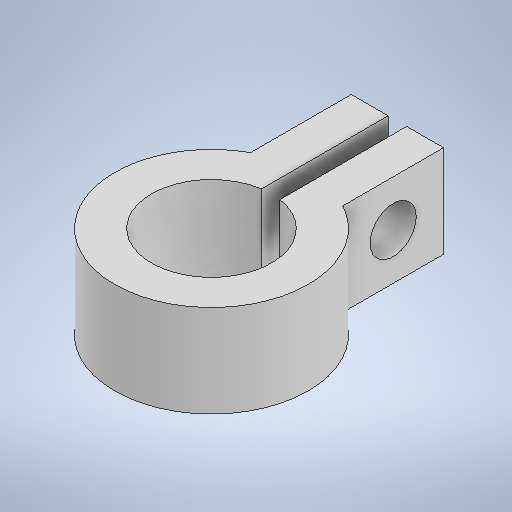
# Autodesk Inventor part: clamp
Saved by Autodesk Inventor 2025 (Build 290162010, 162A)
## iProperties
Created: 2025-03-23
Part Number: clamp
Material: Generic
Document SubType Name: Modeling
Designer: aduwa
Density: 1 g/cm^3
Appearance: Default
Author: aduwa
Autodesk Inventor part; units mm, degrees
ref_plane "YZ Plane" through (0, 0, 0) normal (1, 0, 0) x (0, 1, 0)
ref_plane "XZ Plane" through (0, 0, 0) normal (0, 1, 0) x (-1, 0, 0)
ref_plane "XY Plane" through (0, 0, 0) normal (0, 0, 1) x (1, 0, 0)
sketch "Sketch1" plane through (0, 0, 0) normal (0, 1, 0) x (-1, 0, 0)
  circle A0 centre (0, 0) radius 3.25
  circle A1 centre (0, 0) radius 5.25
  line L0 (0.5, -3.2113) -> (0.5, -10.0767)
  line L1 (0.5, -10.0767) -> (2.5, -10.0767)
  line L2 (2.5, -10.0767) -> (2.5, -2.0767)
  line L3 (0, 0) -> (0, -1.3981)
  line L4 (-0.5, -3.2113) -> (-0.5, -10.0767)
  line L5 (-0.5, -10.0767) -> (-2.5, -10.0767)
  line L6 (-2.5, -10.0767) -> (-2.5, -2.0767)
  point P0 (0, -5.25)
  point P1 (2.5, -4.6165)
  point P2 (-2.5, -4.6165)
  dimension "d1" = 10.5
  dimension "d0" = 6.5
  dimension "d6" = 0.5
  dimension "d7" = 2
  dimension "d8" = 8
  constraints: 14 end point, 4 symmetric about line, 2 coincident, 2 point on circle, 1 centre point, 1 parallel, 1 vertical, 3 other
  measures "d0" diameter of A0
  measures "d6" distance from line of point (0, 0) L0
  measures "d7" distance of L0.end L1.end
  measures "d8" distance of L1.end L2.end
extrude "Extrusion1" add sketch "Sketch1" along normal blind 5 contours A0 L6 A1 L2 | A0 L4 A1 L6 | L2 A1 L0 A0 | A1 L4 L5 L6 | L2 L1 L0 A1
sketch "Sketch2" plane through (-2.5, 0, -10.0767) normal (-1, 0, 0) x (0, 0, 1)
  line L0 (0, 0) -> (5.4601, 0) projected
  line L1 (5.4601, 0) -> (5.4601, 5) projected
  line L2 (0, 5) -> (5.4601, 5) projected
  line L3 (0, 0) -> (0, 5) projected
  circle A0 centre (2.7301, 2.5) radius 1.25
  point P0 (10.0767, 0)
  point P1 (0, 2.5)
  point P2 (2.7301, 0)
  dimension "d11" = 2.5
  constraints: 2 midpoint, 1 centre point, 1 horizontal alignment, 1 vertical alignment
  measures "d11" diameter of A0
extrude "Extrusion2" cut sketch "Sketch2" against normal through all contours A0
body "Solid1"
